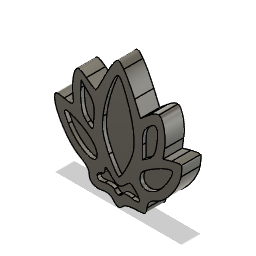
Fungus Counter (Autodesk Fusion 360 design; units mm, degrees)
Autodesk Fusion 360 part; units mm, degrees
note: some values were not read from the file. Set by a fixed rule: which sketch regions a step uses.
sketch "Sketch1" plane through (0, 0, 0) normal (0, 0, 1) x (1, 0, 0)
  spline S0 degree 3 poles (6.0618, -12.8193) (5.8395, -12.5515) (5.4666, -12.4461) (5.0822, -12.5426) knots 0 0 0 0 1 1 1 1
  spline S1 degree 3 poles (5.0822, -12.5426) (4.191, -12.7663) (3.5883, -12.455) (3.5874, -11.7707) knots 0 0 0 0 1 1 1 1
  spline S2 degree 3 poles (3.5874, -11.7707) (3.5869, -11.3694) (3.2527, -10.9997) (2.5517, -10.6252) knots 0 0 0 0 1 1 1 1
  spline S3 degree 3 poles (2.5517, -10.6252) (1.4412, -10.0319) (0.0119, -7.8178) (0.0003, -6.6727) knots 0 0 0 0 1 1 1 1
  spline S4 degree 3 poles (0.0003, -6.6727) (-0.0056, -6.0937) (0.0806, -6.0543) (0.9839, -6.2238) knots 0 0 0 0 1 1 1 1
  spline S5 degree 3 poles (0.9839, -6.2238) (1.9426, -6.4037) (1.9719, -6.3844) (1.9099, -5.6142) knots 0 0 0 0 1 1 1 1
  spline S6 degree 3 poles (1.9099, -5.6142) (1.8113, -4.3896) (1.9122, -3.4768) (2.1958, -3.0284) knots 0 0 0 0 1 1 1 1
  spline S7 degree 3 poles (2.1958, -3.0284) (2.416, -2.6801) (2.5758, -2.7104) (3.2863, -3.2357) knots 0 0 0 0 1 1 1 1
  spline S8 degree 3 poles (3.2863, -3.2357) (3.7441, -3.5742) (4.1769, -3.8512) (4.2479, -3.8512) knots 0 0 0 0 1 1 1 1
  spline S9 degree 3 poles (4.2479, -3.8512) (4.319, -3.8512) (4.6899, -3.198) (5.0722, -2.3996) knots 0 0 0 0 1 1 1 1
  spline S10 degree 3 poles (5.0722, -2.3996) (5.4544, -1.6013) (5.9675, -0.6992) (6.2122, -0.3951) knots 0 0 0 0 1 1 1 1
  spline S11 degree 3 poles (6.2122, -0.3951) (6.6535, 0.1533) (6.6616, 0.1522) (7.1909, -0.5333) knots 0 0 0 0 1 1 1 1
  spline S12 degree 3 poles (7.1909, -0.5333) (7.4844, -0.9135) (7.9962, -1.8717) (8.3283, -2.6626) knots 0 0 0 0 1 1 1 1
  line L0 (8.3283, -2.6626) -> (8.932, -4.1007)
  line L1 (8.932, -4.1007) -> (9.751, -3.4115)
  spline S13 degree 3 poles (9.751, -3.4115) (10.2015, -3.0325) (10.7031, -2.7667) (10.8657, -2.8209) knots 0 0 0 0 1 1 1 1
  spline S14 degree 3 poles (10.8657, -2.8209) (11.3222, -2.9731) (11.632, -4.4296) (11.4498, -5.5663) knots 0 0 0 0 1 1 1 1
  line L2 (11.4498, -5.5663) -> (11.2856, -6.5902)
  line L3 (11.2856, -6.5902) -> (12.188, -6.3314)
  spline S15 degree 3 poles (12.188, -6.3314) (12.6844, -6.189) (13.1447, -6.1269) (13.2111, -6.1932) knots 0 0 0 0 1 1 1 1
  spline S16 degree 3 poles (13.2111, -6.1932) (13.2774, -6.2596) (13.2516, -6.7404) (13.1538, -7.2618) knots 0 0 0 0 1 1 1 1
  spline S17 degree 3 poles (13.1538, -7.2618) (12.9142, -8.5392) (11.5864, -10.3136) (10.5484, -10.7436) knots 0 0 0 0 1 1 1 1
  spline S18 degree 3 poles (10.5484, -10.7436) (9.9523, -10.9905) (9.6774, -11.3106) (9.6176, -11.8273) knots 0 0 0 0 1 1 1 1
  spline S19 degree 3 poles (9.6176, -11.8273) (9.5429, -12.4729) (9.4106, -12.5606) (8.5129, -12.5606) knots 0 0 0 0 1 1 1 1
  spline S20 degree 3 poles (8.5129, -12.5606) (7.952, -12.5606) (7.3361, -12.7162) (7.1443, -12.9062) knots 0 0 0 0 1 1 1 1
  spline S21 degree 3 poles (7.1443, -12.9062) (6.6886, -13.3577) (6.4958, -13.3422) (6.0618, -12.8194) knots 0 0 0 0 1 1 1 1
  line L4 (6.0618, -12.8194) -> (6.0618, -12.8193)
  spline S22 degree 3 poles (7.0543, -11.8532) (7.158, -11.6853) (7.5776, -11.6357) (8.0383, -11.7369) knots 0 0 0 0 1 1 1 1
  spline S23 degree 3 poles (8.0383, -11.7369) (8.9615, -11.9397) (9.0928, -11.5677) (8.3576, -10.8326) knots 0 0 0 0 1 1 1 1
  spline S24 degree 3 poles (8.3576, -10.8326) (7.8968, -10.3717) (7.8507, -10.3717) (7.3899, -10.8326) knots 0 0 0 0 1 1 1 1
  spline S25 degree 3 poles (7.3899, -10.8326) (6.7591, -11.4634) (6.4924, -11.4429) (5.8108, -10.7113) knots 0 0 0 0 1 1 1 1
  spline S26 degree 3 poles (5.8108, -10.7113) (5.3363, -10.202) (5.2471, -10.1801) (5.2471, -10.5731) knots 0 0 0 0 1 1 1 1
  spline S27 degree 3 poles (5.2471, -10.5731) (5.2471, -10.8298) (5.0605, -11.0399) (4.8324, -11.0399) knots 0 0 0 0 1 1 1 1
  spline S28 degree 3 poles (4.8324, -11.0399) (4.6043, -11.0399) (4.4176, -11.2364) (4.4176, -11.4766) knots 0 0 0 0 1 1 1 1
  spline S29 degree 3 poles (4.4176, -11.4766) (4.4176, -11.8148) (4.5988, -11.8735) (5.2208, -11.7369) knots 0 0 0 0 1 1 1 1
  spline S30 degree 3 poles (5.2208, -11.7369) (5.6815, -11.6358) (6.101, -11.6853) (6.2048, -11.8532) knots 0 0 0 0 1 1 1 1
  spline S31 degree 3 poles (6.2048, -11.8532) (6.3043, -12.0142) (6.4954, -12.1459) (6.6295, -12.1459) knots 0 0 0 0 1 1 1 1
  spline S32 degree 3 poles (6.6295, -12.1459) (6.7637, -12.1459) (6.9548, -12.0142) (7.0543, -11.8532) knots 0 0 0 0 1 1 1 1
  spline S33 degree 3 poles (7.648, -8.9332) (8.2347, -7.6516) (8.3343, -7.1043) (8.2168, -5.8082) knots 0 0 0 0 1 1 1 1
  spline S34 degree 3 poles (8.2168, -5.8082) (8.077, -4.2668) (7.0401, -1.3628) (6.6295, -1.3628) knots 0 0 0 0 1 1 1 1
  spline S35 degree 3 poles (6.6295, -1.3628) (6.2163, -1.3628) (5.1816, -4.2715) (5.0402, -5.8309) knots 0 0 0 0 1 1 1 1
  spline S36 degree 3 poles (5.0402, -5.8309) (4.9177, -7.1821) (5.0098, -7.6583) (5.6447, -8.956) knots 0 0 0 0 1 1 1 1
  spline S37 degree 3 poles (5.6447, -8.956) (6.0567, -9.798) (6.5159, -10.487) (6.6652, -10.487) knots 0 0 0 0 1 1 1 1
  spline S38 degree 3 poles (6.6652, -10.487) (6.8145, -10.487) (7.2567, -9.7878) (7.648, -8.9332) knots 0 0 0 0 1 1 1 1
  spline S39 degree 3 poles (4.4176, -9.6575) (4.4176, -8.9539) (3.5284, -8.0609) (2.3286, -7.5596) knots 0 0 0 0 1 1 1 1
  spline S40 degree 3 poles (2.3286, -7.5596) (0.8855, -6.9566) (0.7369, -7.0783) (1.4237, -8.3003) knots 0 0 0 0 1 1 1 1
  spline S41 degree 3 poles (1.4237, -8.3003) (2.3623, -9.9704) (4.4176, -10.9021) (4.4176, -9.6575) knots 0 0 0 0 1 1 1 1
  spline S42 degree 3 poles (10.8995, -9.56) (11.7271, -8.7324) (12.5495, -7.1691) (12.1572, -7.1691) knots 0 0 0 0 1 1 1 1
  spline S43 degree 3 poles (12.1572, -7.1691) (11.5657, -7.1691) (9.1817, -8.5397) (9.0142, -8.9761) knots 0 0 0 0 1 1 1 1
  spline S44 degree 3 poles (9.0142, -8.9761) (8.4931, -10.334) (9.7395, -10.72) (10.8995, -9.56) knots 0 0 0 0 1 1 1 1
  line L5 (3.4669, -4.4338) -> (2.7587, -3.7255)
  line L6 (2.7587, -3.7255) -> (2.7294, -4.4105)
  spline S45 degree 3 poles (2.7294, -4.4105) (2.6591, -6.0547) (2.8321, -6.779) (3.4018, -7.2246) knots 0 0 0 0 1 1 1 1
  spline S46 degree 3 poles (3.4018, -7.2246) (3.9984, -7.6913) (4.0035, -7.6853) (4.089, -6.4184) knots 0 0 0 0 1 1 1 1
  spline S47 degree 3 poles (4.089, -6.4184) (4.161, -5.3521) (4.0586, -5.0255) (3.4669, -4.4338) knots 0 0 0 0 1 1 1 1
  spline S48 degree 3 poles (10.6259, -5.6368) (10.8703, -4.0075) (10.6164, -3.6458) (9.78, -4.4316) knots 0 0 0 0 1 1 1 1
  spline S49 degree 3 poles (9.78, -4.4316) (9.2581, -4.9219) (9.118, -5.3374) (9.118, -6.3942) knots 0 0 0 0 1 1 1 1
  line L7 (9.118, -6.3942) -> (9.118, -7.7348)
  line L8 (9.118, -7.7348) -> (9.7797, -7.3013)
  spline S50 degree 3 poles (9.7797, -7.3013) (10.245, -6.9964) (10.4961, -6.5024) (10.6259, -5.6368) knots 0 0 0 0 1 1 1 1
extrude "Extrude1" add sketch "Sketch1" along normal mid plane 2
extrude "Extrude2" add sketch "Sketch1" along normal mid plane 1.2 contours S22 S23 S24 S25 S26 S27 S28 S29 S30 S31 S32 | S33 S34 S35 S36 S37 S38 | S39 S40 S41 | S42 S43 S44 | L5 L6 S45 S46 S47 | S48 S49 L7 L8 S50
